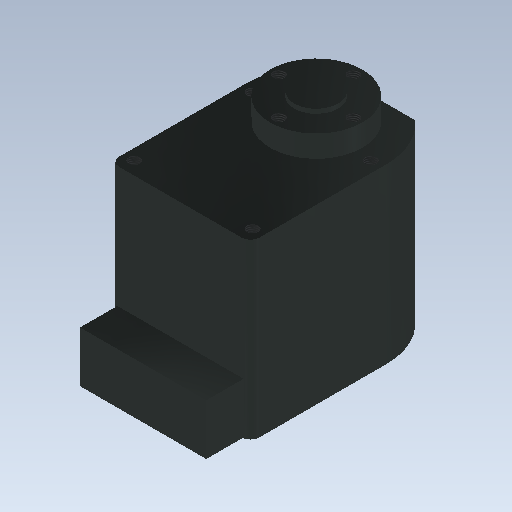
# Autodesk Inventor part: B3M1170
Saved by Autodesk Inventor 2020 (Build 240168000, 168)
## iProperties
Created: 2015-05-21
Part Number: B3M1170
Material: アルミニウム 2014-T4
Document SubType Name: Modeling
Designer: makisumi
Density: 1.84959 g/cm^3
Appearance: ガンメタル - 研磨
Mass: 105 g
Surface Area: 114.821 cm^2
Volume: 56.7692 cm^3
Author: makisumi
Autodesk Inventor part; units mm, degrees
ref_plane "YZ Plane" through (0, 0, 0) normal (1, 0, 0) x (0, 1, 0)
ref_plane "XZ Plane" through (0, 0, 0) normal (0, 1, 0) x (-1, 0, 0)
ref_plane "XY Plane" through (0, 0, 0) normal (0, 0, 1) x (1, 0, 0)
sketch "スケッチ1" plane through (0, 0, 0) normal (0, 1, 0) x (-1, 0, 0)
  line L0 (0, 0) -> (0, -43)
  line L1 (0, -43) -> (32, -43)
  line L2 (32, -43) -> (32, 0)
  line L3 (32, 0) -> (0, 0)
  dimension "d0" = 43
  dimension "d1" = 32
  constraints: 8 end point, 3 perpendicular, 1 vertical
  measures "d0" distance of L0.start L0.end
  measures "d1" distance of L0.end L1.end
extrude "押し出し1" add sketch "スケッチ1" along normal blind 39.5
fillet "フィレット1" radius 2 2 edges at (-32, 19.75, 0) (0, 19.75, 0)
sketch "スケッチ2" plane through (0, 39.5, 0) normal (0, 1, 0) x (1, 0, 0)
  line L0 (0, 43) -> (-32, 43) projected
  line L1 (-16, 43) -> (-16, 0)
  line L2 (-30, 0) -> (-2, 0) projected
  line L3 (-16, 21.5) -> (-16, 3)
  line L4 (-16, 3) -> (-2.5, 3)
  line L5 (0, 2) -> (0, 43) projected
  line L6 (-16, 3) -> (-29.5, 3)
  line L7 (-29.5, 3) -> (-29.5, 30)
  point P0 (0, 0)
  point P1 (-2.5, 30)
  dimension "d5" = 18.5
  dimension "d6" = 13.5
  dimension "d7" = 13.5
  dimension "d8" = 27
  constraints: 10 end point, 3 coincident, 3 midpoint, 1 horizontal, 1 perpendicular, 1 point on line, 1 vertical
  measures "d5" distance of L3.start L3.end
  measures "d6" distance of L3.end L4.end
  measures "d7" distance of L3.end L6.end
  measures "d8" distance of L7.start L7.end
hole "穴1" at (-2.5, 39.5, -3) at (-29.5, 39.5, -3) at (-29.5, 39.5, -30) at (-2.5, 39.5, -30) direction (0, -1, 0) diameter 2.6 end through all
sketch "スケッチ3" plane through (0, 39.5, 0) normal (0, 1, 0) x (1, 0, 0)
  line L0 (0, 43) -> (-32, 43) projected
  line L1 (-16, 43) -> (-16, 0)
  line L2 (-16, 21.5) -> (-16, 31)
  line L3 (-32, 43) -> (-32, 2) projected
  line L4 (-32, 31) -> (-32, 43)
  line L5 (-32, 43) -> (-26.583, 43)
  line L6 (0, 2) -> (0, 43) projected
  line L7 (0, 31) -> (0, 43)
  line L8 (0, 43) -> (-5.417, 43)
  arc A0 (-26.583, 43) -> (-32, 31) centre (-16, 31) ccw
  arc A1 (0, 31) -> (-5.417, 43) centre (-16, 31) ccw
  point P0 (0, 0)
  dimension "d16" = 9.5
  constraints: 12 end point, 5 point on line, 4 point on circle, 2 centre point, 2 collinear, 2 midpoint, 1 coincident, 1 vertical
  measures "d16" distance of L2.start L2.end
extrude "押し出し2" cut sketch "スケッチ3" against normal blind 39.5
sketch "スケッチ4" plane through (0, 39.5, 0) normal (0, 1, 0) x (1, 0, 0)
  arc A0 (-26.583, 43) -> (-32, 31) centre (-16, 31) ccw projected
  circle A1 centre (-16, 31) radius 4
  point P0 (0, 0)
  dimension "d20" = 8
  constraints: 1 centre point, 1 coincident
  measures "d20" diameter of A1
extrude "押し出し3" add sketch "スケッチ4" along normal blind 5
sketch "スケッチ5" plane through (0, 0, 0) normal (0, -1, 0) x (1, 0, 0)
  circle A0 centre (-16, -31) radius 4 projected
  circle A1 centre (-16, -31) radius 4
  point P0 (0, 0)
  constraints: 1 centre point, 1 coincident
extrude "押し出し4" add sketch "スケッチ5" along normal blind 5.5
sketch "スケッチ6" plane through (0, 0, 0) normal (0, -1, 0) x (1, 0, 0)
  line L0 (-30, 0) -> (-2, 0) projected
  line L1 (-16, 0) -> (-1.6, 0)
  line L2 (-1.6, 0) -> (-1.6, 8.5)
  line L3 (-1.6, 0) -> (6.9, 0) construction
  line L4 (-1.6, 8.5) -> (-30.4, 8.5)
  line L5 (-30.4, 8.5) -> (-30.4, -0.1236)
  line L6 (-30.4, -0.1236) -> (-1.6, -0.1236)
  line L7 (-1.6, -0.1236) -> (-1.6, 0)
  point P0 (0, 0)
  dimension "d25" = 14.4
  dimension "d26" = 8.5
  dimension "d27" = 90
  dimension "d28" = 28.8
  constraints: 14 end point, 4 perpendicular, 1 collinear, 1 horizontal, 1 midpoint, 1 parallel, 1 point on line, 1 vertical
  measures "d25" distance of L1.start L1.end
  measures "d26" distance of L1.end L2.end
  measures "d27" angle of L3 L2
  measures "d28" distance of L2.end L4.end
extrude "押し出し5" add sketch "スケッチ6" against normal blind 11.8
sketch "スケッチ7" plane through (0, 0, 0) normal (0, -1, 0) x (1, 0, 0)
  arc A0 (0, -2) -> (-2, 0) centre (-2, -2) ccw projected
  arc A1 (-1.6, -0.0404) -> (-2, 0) centre (-2, -2) ccw
  arc A2 (-30.4, -0.0404) -> (-32, -2) centre (-30, -2) ccw projected
  arc A3 (-30, 0) -> (-30.4, -0.0404) centre (-30, -2) ccw
  line L0 (-1.6, -0.0404) -> (-1.6, 8.5)
  line L1 (-1.6, 8.5) -> (-30.4, 8.5)
  line L2 (-30.4, 8.5) -> (-1.6, 8.5) projected
  line L3 (-30.4, 8.5) -> (-30.4, -0.0404)
  line L4 (-30, 0) -> (-2, 0)
  arc A4 (-30, 0) -> (-30.4, -0.0404) centre (-30, -2) ccw projected
  point P0 (0, 0)
  constraints: 8 end point, 4 point on circle, 2 centre point, 2 coincident, 1 collinear, 1 horizontal, 1 perpendicular, 1 tangent, 1 vertical
extrude "押し出し6" cut sketch "スケッチ7" against normal blind 0.2
thread "ねじ1" size "M2.6x0.45" class "6H" standard "ANSI Metric M Profile" full length
thread "ねじ2" size "M2.6x0.45" class "6H" standard "ANSI Metric M Profile" full length
thread "ねじ3" size "M2.6x0.45" class "6H" standard "ANSI Metric M Profile" full length
thread "ねじ4" size "M2.6x0.45" class "6H" standard "ANSI Metric M Profile" full length
sketch "スケッチ12" plane through (-16, 45, -31) normal (0, 1, 0) x (1, 0, 0)
  circle A0 centre (0, 0) radius 10.5
  point P0 (16, -31)
  dimension "d66" = 21
  constraints: 1 centre point
  measures "d66" diameter of A0
extrude "押し出し9" add sketch "スケッチ12" against normal blind 5
sketch "スケッチ13" plane through (-16, 45, -31) normal (0, 1, 0) x (1, 0, 0)
  circle A0 centre (0, 0) radius 5
  point P0 (16, -31)
  dimension "d69" = 10
  constraints: 1 centre point
  measures "d69" diameter of A0
extrude "押し出し10" add sketch "スケッチ13" along normal blind 1
sketch "スケッチ14" plane through (-16, 45, -31) normal (0, 1, 0) x (1, 0, 0)
  circle A0 centre (0, 0) radius 8.5
  circle A1 centre (0, 8.5) radius 1.3
  circle A2 centre (-8.5, 0) radius 1.3
  circle A3 centre (8.5, 0) radius 1.3
  circle A4 centre (0, -8.5) radius 1.3
  point P0 (16, -31)
  dimension "d72" = 17
  dimension "d73" = 2.6
  dimension "d74" = 2.6
  dimension "d75" = 2.6
  dimension "d76" = 2.6
  constraints: 5 centre point, 4 point on circle
  measures "d72" diameter of A0
  measures "d73" diameter of A1
  measures "d74" diameter of A2
  measures "d75" diameter of A3
  measures "d76" diameter of A4
extrude "押し出し11" cut sketch "スケッチ14" against normal blind 5 contours A0 A3 | A0 A3 | A1 A0 | A0 A1 | A4 A0 | A0 A4 | A2 A0 | A0 A2
thread "ねじ9" size "M2.6x0.45" class "6H" standard "ANSI Metric M Profile" full length
thread "ねじ10" size "M2.6x0.45" class "6H" standard "ANSI Metric M Profile" full length
thread "ねじ11" size "M2.6x0.45" class "6H" standard "ANSI Metric M Profile" full length
thread "ねじ12" size "M2.6x0.45" class "6H" standard "ANSI Metric M Profile" full length
sketch "スケッチ15" plane through (0, 0, 0) normal (0, -1, 0) x (1, 0, 0)
  circle A0 centre (-16, -31) radius 4 projected
  circle A1 centre (-16, -31) radius 6
  point P0 (0, 0)
  dimension "d87" = 12
  constraints: 1 centre point, 1 coincident
  measures "d87" diameter of A1
extrude "押し出し12" add sketch "スケッチ15" along normal blind 1.8
sketch "スケッチ16" plane through (-16, -5.5, -31) normal (0, -1, 0) x (1, 0, 0)
  point P0 (16, 31)
  point P1 (0, 0)
hole "穴3" at (-16, -5.5, -31) direction (0, 1, 0) diameter 3 depth 8 tip angle 118
thread "ねじ13" size "M3x0.5" class "6H" standard "ANSI Metric M Profile" full length
